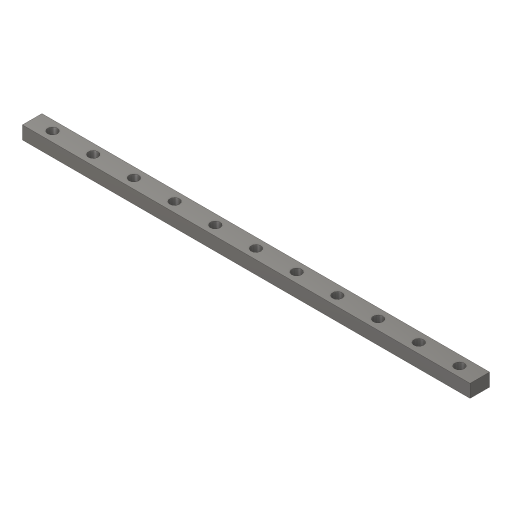
# Autodesk Inventor part: MGNR12_500mm
Saved by Autodesk Inventor 2023.2 (Build 272271000, 271)
## iProperties
Created: 2020-05-08
Part Number: MGNR12_500mm
Material: Stainless Steel
Document SubType Name: Modeling
Designer: Remo
Density: 8 g/cm^3
Appearance: Semi-Polished
Mass: 358.255 g
Surface Area: 222.733 cm^2
Volume: 44.7818 cm^3
Description: HIWIN MGNR12 Linear Rail
Author: Remo
Autodesk Inventor part; units mm, degrees
ref_plane "YZ Plane" through (0, 0, 0) normal (1, 0, 0) x (0, 1, 0)
ref_plane "XZ Plane" through (0, 0, 0) normal (0, 1, 0) x (-1, 0, 0)
ref_plane "XY Plane" through (0, 0, 0) normal (0, 0, 1) x (1, 0, 0)
sketch "Sketch1" plane through (0, 0, 0) normal (1, 0, 0) x (0, 1, 0)
  line L0 (-6, -4) -> (6, -4)
  line L1 (6, -4) -> (6, 4)
  line L2 (6, 4) -> (-6, 4)
  line L3 (-6, 4) -> (-6, -4)
  line L4 (-6, -4) -> (6, 4) construction
  line L5 (6, -4) -> (-6, 4) construction
  point P0 (0, 0)
  dimension "d0" = 12
  dimension "d1" = 8
  constraints: 12 end point, 2 midpoint, 2 parallel, 1 horizontal, 1 perpendicular
  measures "d0" distance of L0.start L0.end
  measures "d1" distance of L2.end L0.start
extrude "Extrusion1" add sketch "Sketch1" along normal blind 275
sketch "Sketch2" plane through (0, -6, 4) normal (0, 0, 1) x (1, 0, 0)
  line L0 (0, 12) -> (0, 0) projected
  line L1 (0, 0) -> (275, 0) projected
  line L2 (275, 12) -> (275, 0) projected
  line L3 (0, 12) -> (275, 12) projected
  point P0 (0, 6)
  point P1 (12.5, 6)
  point P2 (37.5, 6)
  point P3 (62.5, 6)
  point P4 (87.5, 6)
  point P5 (112.5, 6)
  point P6 (137.5, 6)
  point P7 (162.5, 6)
  point P8 (187.5, 6)
  point P9 (212.5, 6)
  point P10 (237.5, 6)
  point P11 (262.5, 6)
  point P12 (287.5, 6)
  point P13 (312.5, 6)
  point P14 (337.5, 6)
  point P15 (362.5, 6)
  point P16 (387.5, 6)
  point P17 (412.5, 6)
  point P18 (437.5, 6)
  point P19 (462.5, 6)
  point P20 (487.5, 6)
  dimension "d6" = 25
  dimension "d11" = 12.5
  dimension "d12" = 6
  constraints: 1 horizontal, 19 other
  measures "d6" distance of point (12.5, 6) point (37.5, 6)
  measures "d11" distance from line of L0 point (12.5, 6)
  measures "d12" distance from line of L1 point (487.5, 6)
hole "Hole1" at (12.5, 0, 4) at (37.5, 0, 4) at (62.5, 0, 4) at (87.5, 0, 4) at (112.5, 0, 4) at (137.5, 0, 4) at (162.5, 0, 4) at (187.5, 0, 4) at (212.5, 0, 4) at (237.5, 0, 4) at (262.5, 0, 4) at (287.5, 0, 4) at (312.5, 0, 4) at (337.5, 0, 4) at (362.5, 0, 4) at (387.5, 0, 4) at (412.5, 0, 4) at (437.5, 0, 4) at (462.5, 0, 4) at (487.5, 0, 4) direction (0, 0, -1) diameter 3.5 depth 8 tip angle 118 counterbore diameter 6 counterbore depth 4.5
equation "\"d11\" = 0.5 * d6"
body "Solid1"
